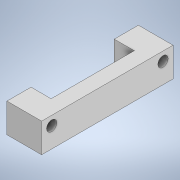
# Autodesk Inventor part: arduino_clamp
Saved by Autodesk Inventor 2022 (Build 260153000, 153)
## iProperties
Created: 2022-01-21
Part Number: arduino_clamp
Material: Generic
Document SubType Name: Modeling
Designer: kylem
Density: 1 g/cm^3
Appearance: Default
Author: kylem
Autodesk Inventor part; units mm, degrees
ref_plane "YZ Plane" through (0, 0, 0) normal (1, 0, 0) x (0, 1, 0)
ref_plane "XZ Plane" through (0, 0, 0) normal (0, 1, 0) x (-1, 0, 0)
ref_plane "XY Plane" through (0, 0, 0) normal (0, 0, 1) x (1, 0, 0)
sketch "Sketch1" plane through (0, 0, 0) normal (1, 0, 0) x (0, 1, 0)
  line L0 (0, 0) -> (4, 0)
  line L1 (4, 0) -> (4, -18)
  line L2 (4, -18) -> (0, -18)
  line L3 (0, -18) -> (0, 0)
  dimension "d0" = 4
  dimension "d1" = 18
  constraints: 8 end point, 2 parallel, 1 horizontal, 1 perpendicular
  measures "d0" distance of L1.end L2.end
  measures "d1" distance of L0.end L1.end
extrude "Extrusion1" add sketch "Sketch1" along normal blind 2.75
sketch "Sketch2" plane through (2.75, 0, 0) normal (1, 0, 0) x (0, 0, -1)
  line L0 (0, 4) -> (0, 0) projected
  line L1 (0, 0) -> (18, 0) projected
  line L2 (0, 4) -> (3.3, 4)
  line L3 (3.3, 4) -> (3.3, 0)
  line L4 (3.3, 0) -> (0, 0)
  line L5 (0, 0) -> (0, 4)
  line L6 (18, 0) -> (18, 4) projected
  line L7 (18, 4) -> (0, 4) projected
  line L8 (18, 0) -> (14.7, 0)
  line L9 (14.7, 0) -> (14.7, 4)
  line L10 (14.7, 4) -> (18, 4)
  line L11 (18, 4) -> (18, 0)
  line L12 (3.3, 4) -> (14.7, 4)
  line L13 (14.7, 4) -> (14.7, 0)
  line L14 (14.7, 0) -> (3.3, 0)
  line L15 (3.3, 0) -> (3.3, 4)
  dimension "d4" = 3.3
  dimension "d5" = 3.3
  constraints: 24 end point, 6 parallel, 3 horizontal, 3 perpendicular, 2 point on line
  measures "d4" distance of L3.end L4.end
  measures "d5" distance of L9.end L10.end
extrude "Extrusion2" cut sketch "Sketch2" against normal blind 2.75 contours L7 L9 L1 L3
sketch "Sketch3" plane through (2.75, 0, 0) normal (1, 0, 0) x (0, 0, -1)
  line L0 (18, 4) -> (14.7, 4) projected
  line L1 (0, 0) -> (18, 0)
  line L2 (18, 0) -> (18, 4)
  line L3 (18, 4) -> (0, 4)
  line L4 (0, 4) -> (0, 0)
  constraints: 8 end point, 2 parallel, 1 horizontal, 1 perpendicular
extrude "Extrusion3" add sketch "Sketch3" along normal blind 2
sketch "Sketch4" plane through (4.75, 0, 0) normal (1, 0, 0) x (0, 0, -1)
  line L0 (3.3, 4) -> (0, 4) projected
  line L1 (0, 4) -> (1.38, 4)
  line L2 (1.38, 4) -> (1.38, 2.76)
  line L3 (18, 4) -> (14.7, 4) projected
  line L4 (18, 4) -> (16.62, 4)
  line L5 (16.62, 4) -> (16.62, 2.76)
  circle A0 centre (1.38, 2.76) radius 0.7
  circle A1 centre (16.62, 2.76) radius 0.7
  point P0 (0, 0)
  dimension "d10" = 1.38
  dimension "d11" = 1.24
  dimension "d12" = 1.38
  dimension "d13" = 1.24
  dimension "d14" = 1.4
  dimension "d15" = 1.4
  constraints: 8 end point, 2 centre point, 2 coincident, 2 perpendicular, 2 point on line
  measures "d10" distance of L0.end L1.end
  measures "d11" distance of L1.end L2.end
  measures "d12" distance of L3.start L4.end
  measures "d13" distance of L4.end L5.end
  measures "d14" diameter of A0
  measures "d15" diameter of A1
extrude "Extrusion4" cut sketch "Sketch4" against normal blind 20
body "Solid1"
